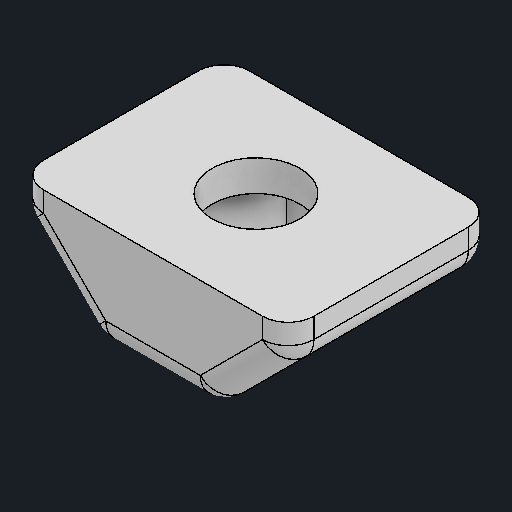
# Autodesk Inventor part: T Nut Adapter
Saved by Autodesk Inventor 2026.2 (Build 302298000, 298)
## iProperties
Created: 2026-07-18
Part Number: T Nut Adapter
Material: Generic
Document SubType Name: Modeling
Designer: JoshuaEah
Density: 1 g/cm^3
Appearance: Default
Author: JoshuaEah
Autodesk Inventor part; units mm, degrees
ref_plane "YZ Plane" through (0, 0, 0) normal (1, 0, 0) x (0, 1, 0)
ref_plane "XZ Plane" through (0, 0, 0) normal (0, 1, 0) x (-1, 0, 0)
ref_plane "XY Plane" through (0, 0, 0) normal (0, 0, 1) x (1, 0, 0)
sketch "Sketch1" plane through (0, 0, 0) normal (0, 1, 0) x (-1, 0, 0)
  line L0 (1.6166, 2.8) -> (3.2332, 0)
  line L1 (3.2332, 0) -> (1.6166, -2.8)
  line L2 (1.6166, -2.8) -> (-1.6166, -2.8)
  line L3 (-1.6166, -2.8) -> (-3.2332, 0)
  line L4 (-3.2332, 0) -> (-1.6166, 2.8)
  line L5 (-1.6166, 2.8) -> (1.6166, 2.8)
  line L6 (5.25, -4) -> (-5.25, -4)
  line L7 (-5.25, -4) -> (-5.25, 4)
  line L8 (-5.25, 4) -> (5.25, 4)
  line L9 (5.25, 4) -> (5.25, -4)
  line L10 (5.25, -4) -> (-5.25, 4) construction
  line L11 (-5.25, -4) -> (5.25, 4) construction
  point P0 (0, 0)
  point P1 (0, 0)
  point P2 (0, 0)
  dimension "d1" = 5.6
  dimension "d2" = 10.5
  dimension "d3" = 8
  constraints: 24 end point, 2 coincident, 2 horizontal, 2 midpoint, 2 parallel, 1 perpendicular, 13 other
  measures "d1" distance between parallel lines of L5 L2
  measures "d2" distance of L7.end L8.end
  measures "d3" distance of L6.end L7.end
extrude "Extrusion1" add sketch "Sketch1" along normal blind 1.2 contours L0 L1 L2 L3 L4 L5 | L6 L7 L8 L9
sketch "Sketch2" plane through (-5.25, 0, 4) normal (0, 0, 1) x (1, 0, 0)
  line L0 (0, 0) -> (10.5, 0) projected
  line L1 (0, 0) -> (3, -3)
  line L2 (3, -3) -> (7.5, -3)
  line L3 (7.5, -3) -> (10.5, 0)
  point P0 (5.25, -3)
  point P1 (5.25, 0)
  dimension "d6" = 45
  dimension "d7" = 3
  constraints: 6 end point, 2 midpoint, 1 horizontal, 1 vertical alignment
  measures "d6" angle of L2 L1
  measures "d7" distance between parallel lines of L2 L0
extrude "Extrusion2" add sketch "Sketch2" against normal up to surface (8 mm away)
extrude "Extrusion3" cut sketch "Sketch1" against normal up to surface (3 mm away) contours L0 L1 L2 L3 L4 L5
fillet "Fillet1" radius 1 6 edges at (5.25, 0, 0) (-5.25, 0, 0) (-2.25, -3, 2.8514) (2.25, -3, 2.8514) (2.25, -3, -2.8514) (-2.25, -3, -2.8514)
fillet "Fillet2" radius 1 18 edges at (2.2185, -2.9239, 4) (3.75, -1.5, 4) (5.1739, 0.0315, 4) (5.25, 0.8071, 4) (-2.2185, -2.9239, 4) (-3.75, -1.5, 4) (-5.1739, 0.0315, 4) (-5.25, 0.8071, 4) (0, -3, 4) (2.2185, -2.9239, -4) (3.75, -1.5, -4) (5.1739, 0.0315, -4) (5.25, 0.8071, -4) (-2.2185, -2.9239, -4) (-3.75, -1.5, -4) (-5.1739, 0.0315, -4) (-5.25, 0.8071, -4) (0, -3, -4)
hole "Hole1" at (0, 0, 0) direction (0, 1, 0) diameter 3.4036 end through all clearance for "Socket Head Cap Screw" size "M3" standard "Ansi Metric M Profile"
body "Solid1"
